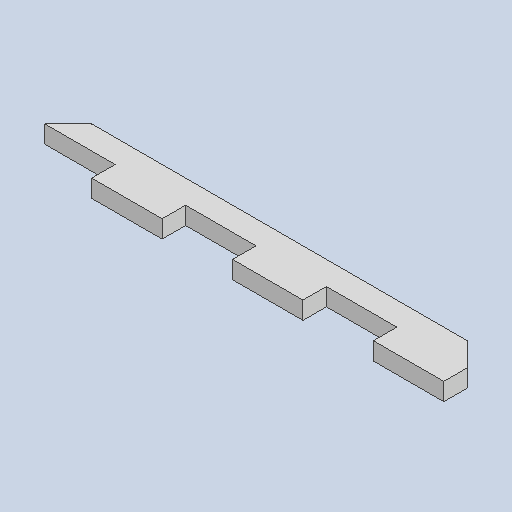
# Autodesk Inventor part: креп
Saved by Autodesk Inventor 2023.1 (Build 271208000, 208)
## iProperties
Created: 2025-01-21
Part Number: креп
Material: Типовые
Document SubType Name: Modeling
Designer: DELL
Density: 1 g/cm^3
Appearance: По умолчанию
Author: DELL
Autodesk Inventor part; units mm, degrees
ref_plane "YZ Plane" through (0, 0, 0) normal (1, 0, 0) x (0, 1, 0)
ref_plane "XZ Plane" through (0, 0, 0) normal (0, 1, 0) x (-1, 0, 0)
ref_plane "XY Plane" through (0, 0, 0) normal (0, 0, 1) x (1, 0, 0)
sketch "Эскиз1" plane through (0, 0, 0) normal (0, 1, 0) x (-1, 0, 0)
  line L0 (0, 4) -> (0, 0)
  line L1 (-4, -4) -> (-68, -4)
  line L2 (-72, 0) -> (-72, 4)
  line L3 (-72, 0) -> (-68.5995, -3.4005)
  line L4 (-72, 0) -> (-67.191, 0) construction
  line L5 (-68.5995, -3.4005) -> (-68, -4)
  line L6 (0, 0) -> (-3.643, -3.643)
  line L7 (0, 0) -> (5.152, 0) construction
  line L8 (-3.643, -3.643) -> (-4, -4)
  line L9 (-48, 4) -> (-48, 0)
  line L10 (-48, 4) -> (-48, 0)
  line L11 (-24, 4) -> (-24, 0)
  line L12 (-12, 4) -> (-12, 0)
  line L13 (-36, 4) -> (-36, 0)
  line L14 (-60, 4) -> (-60, 0)
  line L15 (-72, 4) -> (-60, 4)
  line L16 (-48, 4) -> (-36, 4)
  line L17 (-24, 4) -> (-12, 4)
  line L18 (-60, 0) -> (-48, 0)
  line L19 (-36, 0) -> (-24, 0)
  line L20 (-12, 0) -> (0, 0)
  point P0 (0, 0)
  point P1 (0, 2)
  point P2 (-24, 2)
  point P3 (-48, 2)
  point P4 (-72, 2)
  point P5 (-48, 2)
  point P6 (-12, 2)
  point P7 (-36, 2)
  point P8 (-60, 2)
  dimension "d0" = 4
  dimension "d1" = 72
  dimension "d3" = 4.809
  dimension "d4" = 45
  dimension "d5" = 5.152
  dimension "d6" = 135
  dimension "d7" = 24
  dimension "d8" = 24
  dimension "d9" = 24
  dimension "d10" = 12
  dimension "d12" = 12
  dimension "d13" = 12
  constraints: 42 end point, 8 midpoint, 7 parallel, 6 vertical, 5 horizontal, 3 perpendicular, 2 equal length, 2 point on line, 1 coincident
  measures "d0" distance of L2.start L2.end
  measures "d1" distance of L2.end L0.start
  measures "d3" distance of L2.start L3.end
  measures "d4" angle of L3 L4
  measures "d5" distance of L0.end L6.end
  measures "d6" angle of L6 L7
  measures "d7" distance of point (0, 2) point (-24, 2)
  measures "d8" distance of point (-48, 2) point (-24, 2)
  measures "d9" distance of point (-72, 2) point (-48, 2)
  measures "d10" distance of point (-12, 2) point (0, 2)
  measures "d12" distance of point (-24, 2) point (-36, 2)
  measures "d13" distance of point (-60, 2) point (-48, 2)
extrude "Выдавливание1" add sketch "Эскиз1" along normal blind 3
